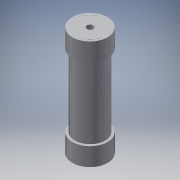
# Autodesk Inventor part: Roller Drum 10-Inch
Saved by Autodesk Inventor 2016 (Build 200138000, 138)
## iProperties
Created: 2016-01-27
Part Number: Roller Drum 10-Inch
Material: PVC-Piping
Document SubType Name: Modeling
Designer: Jack Jaworski
Density: 1.4 g/cm^3
Appearance: Smooth - White
Mass: 414.397 g
Surface Area: 1064.03 cm^2
Volume: 295.998 cm^3
Author: Jack Jaworski
Autodesk Inventor part; units mm, degrees
ref_plane "YZ Plane" through (0, 0, 0) normal (1, 0, 0) x (0, 1, 0)
ref_plane "XZ Plane" through (0, 0, 0) normal (0, 1, 0) x (-1, 0, 0)
ref_plane "XY Plane" through (0, 0, 0) normal (0, 0, 1) x (1, 0, 0)
sketch "Sketch6" plane through (0, 0, 0) normal (0, 1, 0) x (-1, 0, 0)
  circle A0 centre (0, 0) radius 31.75
  circle A1 centre (0, 0) radius 26.5938
  dimension "d16" = 63.5
  dimension "d17" = 5.1562
  constraints: 2 centre point, 2 coincident
  measures "d16" diameter of A0
  measures "d17" radial gap between concentric circles of A0 A1
extrude "Extrusion5" add sketch "Sketch6" along normal blind 190.5
sketch "Sketch7" plane through (0, 0, 0) normal (0, -1, 0) x (1, 0, 0)
  circle A0 centre (0, 0) radius 36.9062
  circle A1 centre (0, 0) radius 31.75
  dimension "d20" = 63.5
  dimension "d21" = 5.1562
  constraints: 2 centre point, 2 coincident
  measures "d20" diameter of A1
  measures "d21" radial gap between concentric circles of A0 A1
extrude "Extrusion6" add sketch "Sketch7" along normal mid plane 38.1
sketch "Sketch8" plane through (0, -19.05, 0) normal (0, -1, 0) x (1, 0, 0)
  circle A0 centre (0, 0) radius 31.75
  constraints: 1 centre point, 1 coincident
extrude "Extrusion7" add sketch "Sketch8" against normal blind 5.1562
sketch "Sketch9" plane through (0, 190.5, 0) normal (0, 1, 0) x (1, 0, 0)
  circle A0 centre (0, 0) radius 31.75
  circle A1 centre (0, 0) radius 36.9062
  constraints: 2 centre point, 2 coincident
extrude "Extrusion8" add sketch "Sketch9" along normal mid plane 38.1
sketch "Sketch10" plane through (0, 209.55, 0) normal (0, 1, 0) x (1, 0, 0)
  circle A0 centre (0, 0) radius 31.7444
  dimension "d28" = 63.4887
  constraints: 1 centre point, 1 coincident
  measures "d28" diameter of A0
extrude "Extrusion9" add sketch "Sketch10" against normal blind 5.1562
sketch "Sketch11" plane through (0, 209.55, 0) normal (0, 1, 0) x (1, 0, 0)
  line L0 (-7.3323, 0) -> (-3.6662, 6.35)
  line L1 (-3.6662, 6.35) -> (3.6662, 6.35)
  line L2 (3.6662, 6.35) -> (7.3323, 0)
  line L3 (7.3323, 0) -> (3.6662, -6.35)
  line L4 (3.6662, -6.35) -> (-3.6662, -6.35)
  line L5 (-3.6662, -6.35) -> (-7.3323, 0)
  point P0 (0, 0)
  point P1 (0, 0)
  dimension "d31" = 12.7
  constraints: 12 end point, 1 coincident, 1 horizontal, 13 other
  measures "d31" distance between parallel lines of L5 L2
extrude "Extrusion10" cut sketch "Sketch11" against normal blind 228.6
body "Solid2"
